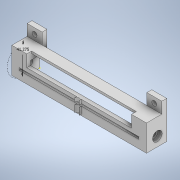
# Autodesk Inventor part: front_2-6
Saved by Autodesk Inventor 2020 (Build 240168000, 168)
## iProperties
Created: 2020-02-06
Part Number: front_2-6
Material: Generic
Document SubType Name: Modeling
Designer: akend
Density: 1 g/cm^3
Appearance: Default
Author: akend
## iProperties of the stored document _3DPrint.ipt
Created: 2020-02-07
Part Number: _3DPrint
Material: Generic
Document SubType Name: Modeling
Designer: akend
Density: 1 g/cm^3
Appearance: Default
Author: akend
Autodesk Inventor part; units mm, degrees
ref_plane "YZ Plane" through (0, 0, 0) normal (1, 0, 0) x (0, 1, 0)
ref_plane "XZ Plane" through (0, 0, 0) normal (0, 1, 0) x (-1, 0, 0)
ref_plane "XY Plane" through (0, 0, 0) normal (0, 0, 1) x (1, 0, 0)
sketch "Sketch1" plane through (0, 0, 0) normal (1, 0, 0) x (0, 1, 0)
  line L0 (0, 0) -> (35, 0)
  line L1 (35, 0) -> (35, 27)
  line L2 (35, 27) -> (0, 27)
  line L3 (0, 27) -> (0, 0)
  line L4 (0, 27) -> (25, 27) construction
  line L5 (25, 27) -> (25, 0) construction
  line L6 (25, 0) -> (0, 0) construction
  line L7 (0, 0) -> (0, 27) construction
  circle A0 centre (12.5, 12.5) radius 6.35
  dimension "d0" = 35
  dimension "d1" = 27
  dimension "d2" = 25
  dimension "d3" = 12.7
  constraints: 16 end point, 4 parallel, 2 horizontal, 2 perpendicular, 1 centre point, 1 coincident, 1 point on line
  measures "d0" distance of L2.end L1.end
  measures "d1" distance of L1.end L0.end
  measures "d2" distance of L5.end L6.end
  measures "d3" diameter of A0
extrude "Extrusion1" add sketch "Sketch1" along normal blind 10
sketch "Sketch2" plane through (10, 0, 0) normal (1, 0, 0) x (0, 0, -1)
  line L0 (0, 35) -> (-27, 35) projected
  line L1 (0, 0) -> (0, 35) projected
  line L2 (-27, 35) -> (0, 35)
  line L3 (0, 35) -> (0, 25)
  line L4 (0, 25) -> (-27, 25)
  line L5 (-27, 25) -> (-27, 35)
  dimension "d6" = 10
  constraints: 8 end point, 2 parallel, 1 horizontal, 1 perpendicular, 1 point on line
  measures "d6" distance of L2.end L3.end
extrude "Extrusion2" add sketch "Sketch2" along normal blind 10
sketch "Sketch3" plane through (10, 0, 0) normal (1, 0, 0) x (0, 0, -1)
  point P0 (0, 0)
sketch "Sketch4" plane through (0, 0, 0) normal (0, 0, -1) x (-1, 0, 0)
  point P0 (0, 0)
sketch "Sketch5" plane through (10, 0, 0) normal (1, 0, 0) x (0, 0, -1)
  point P0 (0, 0)
sketch "Sketch6" plane through (10, 0, 0) normal (1, 0, 0) x (0, 0, -1)
  line L0 (-27, 25) -> (-27, 0) projected
  line L1 (-27, 0) -> (-22, 0)
  line L2 (-22, 0) -> (-22, 11)
  line L3 (-22, 11) -> (-27, 11)
  line L4 (-27, 11) -> (-27, 0)
  line L5 (-22, 14) -> (-27, 14)
  line L6 (-27, 14) -> (-27, 19)
  line L7 (-27, 19) -> (-22, 19)
  line L8 (-22, 19) -> (-22, 14)
  point P0 (0, 0)
  dimension "d9" = 5
  dimension "d10" = 11
  dimension "d11" = 5
  constraints: 16 end point, 4 parallel, 2 horizontal, 2 perpendicular, 2 point on line
  measures "d9" distance of L3.end L2.end
  measures "d10" distance of L2.end L1.end
  measures "d11" distance of L5.end L6.end
extrude "Extrusion3" add sketch "Sketch6" along normal blind 150
sketch "Sketch7" plane through (10, 19, 27) normal (0, 1, 0) x (1, 0, 0)
  line L0 (-10, 0) -> (10, 0) projected
  line L1 (0, 5) -> (150, 5) projected
  line L2 (0, 0) -> (10, 0)
  line L3 (10, 0) -> (10, 5)
  line L4 (10, 5) -> (0, 5)
  line L5 (0, 5) -> (0, 0)
  point P0 (-10, 27)
  dimension "d14" = 10
  constraints: 8 end point, 2 parallel, 1 horizontal, 1 midpoint, 1 perpendicular, 1 point on line
  measures "d14" distance of L4.end L3.end
extrude "Extrusion4" add sketch "Sketch7" along normal blind 7.5
sketch "Sketch8" plane through (160, 0, 0) normal (1, 0, 0) x (0, 0, -1)
  line L0 (-27, 14) -> (-22, 14) projected
  line L1 (-27, 14) -> (-22, 14)
  line L2 (-22, 25) -> (-22, 14) projected
  line L3 (-22, 14) -> (-22, 25)
  line L4 (-22, 25) -> (0, 25) projected
  line L5 (-22, 25) -> (0, 25)
  line L6 (0, 25) -> (0, 35) projected
  line L7 (0, 25) -> (0, 35)
  line L8 (0, 35) -> (-27, 35)
  line L9 (-27, 35) -> (-27, 14)
  line L10 (-22, 11) -> (-22, 0) projected
  line L11 (-27, 0) -> (-22, 0)
  line L12 (-22, 0) -> (-22, 11)
  line L13 (-22, 11) -> (-27, 11)
  line L14 (-27, 11) -> (-27, 0)
  point P0 (0, 0)
  dimension "d9" = 5
  dimension "d10" = 11
  dimension "d11" = 5
  constraints: 20 end point, 5 perpendicular, 4 equal length, 1 horizontal
extrude "Extrusion5" add sketch "Sketch8" along normal blind 10
sketch "Sketch9" plane through (170, 0, 0) normal (1, 0, 0) x (0, 0, -1)
  line L0 (0, 35) -> (-27, 35) projected
  line L1 (-27, 35) -> (0, 35)
  line L2 (0, 35) -> (0, 0)
  line L3 (0, 0) -> (-27, 0)
  line L4 (-27, 0) -> (-27, 35)
  circle A0 centre (-12.5, 12.5) radius 6.35 projected
  circle A1 centre (-12.5, 12.5) radius 6.35
  constraints: 8 end point, 2 parallel, 1 centre point, 1 coincident, 1 horizontal, 1 perpendicular
extrude "Extrusion6" add sketch "Sketch9" along normal blind 10
fillet "Fillet1" radius 2 2 edges at (90, 11, 22) (90, 14, 22)
sketch "Sketch10" plane through (20, 0, 0) normal (1, 0, 0) x (0, 0, -1)
  line L0 (0, 35) -> (-27, 35) projected
  line L1 (-13.5, 35) -> (-20.5, 35)
  line L2 (-20.5, 35) -> (-6.5, 35)
  line L3 (-20.5, 35) -> (-6.5, 35)
  line L4 (-6.5, 35) -> (-6.5, 32)
  line L5 (-6.5, 32) -> (-20.5, 32)
  line L6 (-20.5, 32) -> (-20.5, 35)
  point P0 (0, 0)
  dimension "d22" = 7
  dimension "d23" = 14
  dimension "d24" = 3
  constraints: 12 end point, 2 parallel, 2 point on line, 1 horizontal, 1 midpoint, 1 perpendicular
  measures "d22" distance of L1.start L1.end
  measures "d23" distance of L1.end L2.end
  measures "d24" distance of L3.end L4.end
extrude "Extrusion7" add sketch "Sketch10" along normal blind 140
sketch "Sketch11" plane through (0, 35, 27) normal (0, 1, 0) x (1, 0, 0)
  point P0 (0, 27)
sketch "Sketch12" plane through (160, 25, 0) normal (0, 0, -1) x (-1, 0, 0)
  line L0 (-4, 3.5) -> (-16, 3.5)
  line L1 (-16, 3.5) -> (-16, 6.5)
  line L2 (-16, 6.5) -> (-4, 6.5)
  line L3 (-4, 6.5) -> (-4, 3.5)
  line L4 (-4, 3.5) -> (-16, 6.5) construction
  line L5 (-16, 3.5) -> (-4, 6.5) construction
  line L6 (156, 6.5) -> (144, 6.5)
  line L7 (144, 6.5) -> (144, 3.5)
  line L8 (144, 3.5) -> (156, 3.5)
  line L9 (156, 3.5) -> (156, 6.5)
  line L10 (156, 6.5) -> (144, 3.5) construction
  line L11 (144, 6.5) -> (156, 3.5) construction
  point P0 (160, -25)
  point P1 (-10, 5)
  point P2 (150, 5)
  dimension "d27" = 12
  dimension "d28" = 3
  dimension "d29" = 12
  dimension "d30" = 3
  constraints: 24 end point, 4 midpoint, 4 parallel, 2 horizontal, 2 perpendicular
  measures "d27" distance of L0.start L0.end
  measures "d28" distance of L0.end L1.end
  measures "d29" distance of L6.start L6.end
  measures "d30" distance of L7.end L6.end
extrude "Extrusion8" cut sketch "Sketch12" against normal blind 23.5
sketch "Sketch13" plane through (0, 0, 0) normal (-1, 0, 0) x (0, 0, 1)
  circle A0 centre (12.5, 12.5) radius 6.35 construction
  circle A1 centre (12.5, 12.5) radius 20.6375 construction
  point P0 (0, 0)
  dimension "d33" = 41.275
  constraints: 1 centre point, 1 coincident
  measures "d33" diameter of A1
sketch "Sketch14" plane through (170, 0, 0) normal (-1, 0, 0) x (0, 0, 1)
  circle A0 centre (12.5, 12.5) radius 6.35 projected
  circle A1 centre (12.5, 12.5) radius 6.35
  circle A2 centre (12.5, 12.5) radius 3.5
  point P0 (0, 0)
  dimension "d34" = 7
  constraints: 2 centre point, 2 coincident
  measures "d34" diameter of A2
extrude "Extrusion9" add sketch "Sketch14" against normal blind 4.5
sketch "Sketch15" plane through (10, 0, 0) normal (1, 0, 0) x (0, 0, -1)
  circle A0 centre (-12.5, 12.5) radius 3.5 projected
  circle A1 centre (-12.5, 12.5) radius 6.35
  circle A2 centre (-12.5, 12.5) radius 3.5
  point P0 (0, 0)
  dimension "d37" = 7
  constraints: 2 centre point, 2 coincident
  measures "d37" diameter of A2
extrude "Extrusion10" add sketch "Sketch15" against normal blind 4.5
sketch "Sketch16" plane through (0, 35, 27) normal (0, 1, 0) x (1, 0, 0)
  point P0 (0, 27)
sketch "Sketch17" plane through (20, 19, 27) normal (0, 1, 0) x (1, 0, 0)
  line L0 (-10, 0) -> (150, 0) projected
  circle A0 centre (70, -3.175) radius 3.175
  line L1 (66.825, 0) -> (73.175, 0)
  line L2 (73.175, 0) -> (73.175, -3.175)
  line L3 (73.175, -3.175) -> (66.825, -3.175)
  line L4 (66.825, -3.175) -> (66.825, 0)
  point P0 (-20, 27)
  point P1 (70, 0)
  point P2 (66.825, -3.175)
  point P3 (73.175, 0)
  constraints: 8 end point, 2 parallel, 2 point on circle, 1 centre point, 1 horizontal, 1 midpoint, 1 perpendicular, 1 point on line
extrude "Extrusion11" add sketch "Sketch17" against normal blind 19 contours L0 A0 L4 | L0 L2 A0
sketch "Sketch18" plane through (0, 0, 0) normal (-1, 0, 0) x (0, 0, 1)
  point P0 (0, 0)
sketch "Sketch19" plane through (160, 19, 27) normal (0, 0, 1) x (1, 0, 0)
  line L0 (-150, -8) -> (10, -8) projected
  line L1 (-74.7441, -5.023) -> (-65.8367, -5.023)
  line L2 (-65.8367, -5.023) -> (-65.8367, -8)
  line L3 (-65.8367, -8) -> (-74.7441, -8)
  line L4 (-74.7441, -8) -> (-74.7441, -5.023)
  line L5 (-150, -19) -> (10, -19) projected
  line L6 (-74.2056, -19) -> (-65.8367, -19)
  line L7 (-65.8367, -19) -> (-65.8367, -17)
  line L8 (-65.8367, -17) -> (-74.2056, -17)
  line L9 (-74.2056, -17) -> (-74.2056, -19)
  point P0 (-160, -19)
  dimension "d42" = 2
  constraints: 16 end point, 4 parallel, 3 point on line, 2 horizontal, 2 perpendicular
  measures "d42" distance of L7.end L6.end
extrude "Extrusion12" cut sketch "Sketch19" along normal blind 19
sketch "Sketch20" plane through (0, 35, 27) normal (0, 1, 0) x (1, 0, 0)
  line L0 (0, 0) -> (0, 27) projected
  line L1 (20, 20.5) -> (160, 20.5) projected
  line L2 (0, 27) -> (20, 27)
  line L3 (20, 27) -> (20, 20.5)
  line L4 (20, 20.5) -> (0, 20.5)
  line L5 (0, 20.5) -> (0, 27)
  constraints: 8 end point, 2 parallel, 1 horizontal, 1 perpendicular
extrude "Extrusion13" add sketch "Sketch20" along normal blind 15
sketch "Sketch21" plane through (0, 35, 6.5) normal (0, 0, 1) x (1, 0, 0)
  line L0 (0, 0) -> (20, 0) construction
  line L1 (20, 15) -> (0, 15) construction
  line L2 (0, 0) -> (20, 15) construction
  circle A0 centre (10, 7.5) radius 3.2
  point P0 (0, -35)
  dimension "d47" = 6.4
  constraints: 2 end point, 1 centre point, 1 midpoint
  measures "d47" diameter of A0
extrude "Extrusion14" cut sketch "Sketch21" against normal blind 15
sketch "Sketch22" plane through (160, 25, 0) normal (0, 0, -1) x (-1, 0, 0)
  line L0 (-20, 10) -> (-20, -25) projected
  line L1 (-20, 10) -> (0, 10)
  line L2 (0, 10) -> (0, 25)
  line L3 (0, 25) -> (-20, 25)
  line L4 (-20, 25) -> (-20, 10)
  circle A0 centre (-10, 17.5) radius 3.2
  point P0 (160, -25)
  dimension "d50" = 20
  dimension "d51" = 15
  dimension "d52" = 6.4
  constraints: 8 end point, 2 parallel, 1 centre point, 1 horizontal, 1 perpendicular
  measures "d50" distance of L3.end L2.end
  measures "d51" distance of L2.end L1.end
  measures "d52" diameter of A0
extrude "Extrusion15" add sketch "Sketch22" against normal blind 6.5
body "Solid1"
